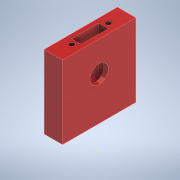
# Autodesk Inventor part: Soporte_Horizontal_Modificado
Saved by Autodesk Inventor 2022 (Build 260153000, 153)
## iProperties
Created: 2022-01-28
Part Number: Soporte_Horizontal_Modificado
Material: ABS Plastic
Document SubType Name: Modeling
Designer: hurta
Density: 1.06 g/cm^3
Appearance: Red
Author: hurta
Autodesk Inventor part; units mm, degrees
ref_plane "YZ Plane" through (0, 0, 0) normal (1, 0, 0) x (0, 1, 0)
ref_plane "XZ Plane" through (0, 0, 0) normal (0, 1, 0) x (-1, 0, 0)
ref_plane "XY Plane" through (0, 0, 0) normal (0, 0, 1) x (1, 0, 0)
sketch "Sketch1" plane through (0, 0, 0) normal (0, 1, 0) x (-1, 0, 0)
  line L0 (45, -30) -> (-45, -30)
  line L1 (-45, -30) -> (-45, 30)
  line L2 (-45, 30) -> (45, 30)
  line L3 (45, 30) -> (45, -30)
  line L4 (45, -30) -> (-45, 30) construction
  line L5 (-45, -30) -> (45, 30) construction
  line L6 (30, -30) -> (-30, -30)
  line L7 (-30, -30) -> (-30, 30)
  line L8 (-30, 30) -> (30, 30)
  line L9 (30, 30) -> (30, -30)
  line L10 (30, -30) -> (-30, 30) construction
  line L11 (-30, -30) -> (30, 30) construction
  point P0 (0, 0)
  point P1 (30, -30)
  point P2 (30, 30)
  dimension "d0" = 90
  dimension "d1" = 60
  dimension "d2" = 60
  constraints: 24 end point, 4 midpoint, 4 parallel, 2 horizontal, 2 perpendicular, 1 point on line
  measures "d0" distance of L1.end L2.end
  measures "d1" distance of L0.end L1.end
  measures "d2" distance of L7.end L8.end
extrude "Extrusion1" add sketch "Sketch1" against normal blind 10 contours L0 L7 L2 L9
extrude "Extrusion2" add sketch "Sketch1" along normal blind 80 and the other way blind 10 contours L0 L9 L2 L3 | L0 L1 L2 L7
sketch "Sketch3" plane through (0, -10, 0) normal (0, -1, 0) x (1, 0, 0)
  point P0 (0, 0)
  point P1 (0, 5)
  point P2 (0, -5)
  dimension "d16" = 5
  dimension "d17" = 5
  constraints: 2 vertical alignment
  measures "d16" distance of point (0, 5) point (0, 0)
  measures "d17" distance of point (0, 0) point (0, -5)
hole "Hole2" at (0, -10, 5) at (0, -10, -5) direction (0, 1, 0) diameter 5.5 end through all clearance for "Hex Head Bolt" size "M5" standard "Ansi Metric M Profile"
sketch "Sketch4" plane through (45, -10, -30) normal (1, 0, 0) x (0, 0, -1)
  circle A0 centre (-30, 65) radius 11
  line L0 (-41, 65) -> (-41, 90)
  line L1 (-60, 90) -> (0, 90) projected
  line L2 (-19, 65) -> (-19, 90)
  circle A1 centre (-30, 65) radius 7.5
  point P0 (-30, 10)
  dimension "d25" = 22
  dimension "d26" = 15
  dimension "d27" = 25
  constraints: 4 end point, 2 centre point, 2 perpendicular, 2 point on circle, 2 point on line, 2 tangent, 1 coincident, 1 vertical alignment
  measures "d25" diameter of A0
  measures "d26" diameter of A1
  measures "d27" distance from line of L1 A0.centre
extrude "Extrusion3" cut sketch "Sketch4" against normal through all contours A1
sketch "Sketch5" plane through (0, 80, 0) normal (0, 1, 0) x (1, 0, 0)
  line L0 (-41.5, 11.25) -> (-33.5, 11.25)
  line L1 (-33.5, 11.25) -> (-33.5, -11.25)
  line L2 (-33.5, -11.25) -> (-41.5, -11.25)
  line L3 (-41.5, -11.25) -> (-41.5, 11.25)
  line L4 (-41.5, 11.25) -> (-33.5, -11.25) construction
  line L5 (-33.5, 11.25) -> (-41.5, -11.25) construction
  line L6 (33.5, 11.25) -> (41.5, 11.25)
  line L7 (41.5, 11.25) -> (41.5, -11.25)
  line L8 (41.5, -11.25) -> (33.5, -11.25)
  line L9 (33.5, -11.25) -> (33.5, 11.25)
  line L10 (33.5, 11.25) -> (41.5, -11.25) construction
  line L11 (41.5, 11.25) -> (33.5, -11.25) construction
  line L12 (-45, 30) -> (-45, -30) projected
  line L13 (-30, 30) -> (-45, 30) projected
  line L14 (45, 30) -> (30, 30) projected
  point P0 (0, 0)
  point P1 (-37.5, 0)
  point P2 (37.5, 0)
  point P3 (-37.5, 0)
  point P4 (37.5, 0)
  point P5 (-37.5, 0)
  point P6 (-45, 0)
  point P7 (-37.5, 30)
  point P8 (-37.5, 11.25)
  point P9 (37.5, 11.25)
  point P10 (37.5, 30)
  dimension "d32" = 8
  dimension "d33" = 22.5
  dimension "d34" = 8
  dimension "d35" = 22.5
  constraints: 24 end point, 12 midpoint, 4 parallel, 2 horizontal, 2 horizontal alignment, 2 perpendicular, 2 vertical alignment
  measures "d32" distance of L1.end L2.end
  measures "d33" distance of L0.end L1.end
  measures "d34" distance of L7.end L8.end
  measures "d35" distance of L6.end L7.end
extrude "Extrusion5" cut sketch "Sketch5" against normal blind 36.75
sketch "Sketch6" plane through (45, -10, -30) normal (1, 0, 0) x (0, 0, -1)
  point P0 (-30, 10)
sketch "Sketch7" plane through (-45, -10, 30) normal (-1, 0, 0) x (0, 0, 1)
  line L0 (-69.6025, -105.0508) -> (27.4472, -105.0508)
  line L1 (27.4472, -105.0508) -> (27.4472, 137.5734)
  line L2 (27.4472, 137.5734) -> (-69.6025, 137.5734)
  line L3 (-69.6025, 137.5734) -> (-69.6025, -105.0508)
  point P0 (-30, 10)
  constraints: 8 end point, 2 parallel, 1 horizontal, 1 perpendicular
extrude "Extrusion6" cut sketch "Sketch7" against normal up to surface (75 mm away)
sketch "Sketch8" plane through (0, -10, 0) normal (0, -1, 0) x (1, 0, 0)
  line L0 (55.2414, 58.8952) -> (10.7003, 58.8952)
  line L1 (10.7003, 58.8952) -> (10.7003, -57.3293)
  line L2 (10.7003, -57.3293) -> (55.2414, -57.3293)
  line L3 (55.2414, -57.3293) -> (55.2414, 58.8952)
  point P0 (0, 0)
  constraints: 8 end point, 2 parallel, 1 horizontal, 1 perpendicular
extrude "Extrusion7" cut sketch "Sketch8" against normal blind 30
sketch "Sketch9" plane through (0, 20, 0) normal (0, -1, 0) x (1, 0, 0)
  line L0 (45, -30) -> (30, -30) projected
  line L1 (30, 30) -> (45, 30) projected
  point P0 (0, 0)
  point P1 (37.5, 15)
  point P2 (37.5, -15)
  point P3 (37.5, -30)
  dimension "d45" = 15
  dimension "d46" = 15
  constraints: 2 vertical alignment, 1 midpoint
  measures "d45" distance from line of point (37.5, 15) L1
  measures "d46" distance from line of point (37.5, -15) L0
hole "Hole3" at (37.5, 20, 15) at (37.5, 20, -15) direction (0, 1, 0) diameter 4.134 end through all thread size "M5x0.8" class "6H" standard "ISO Metric profile"
equation "\"d34\" = d32"
equation "\"d35\" = d33"
body "Solid1"
